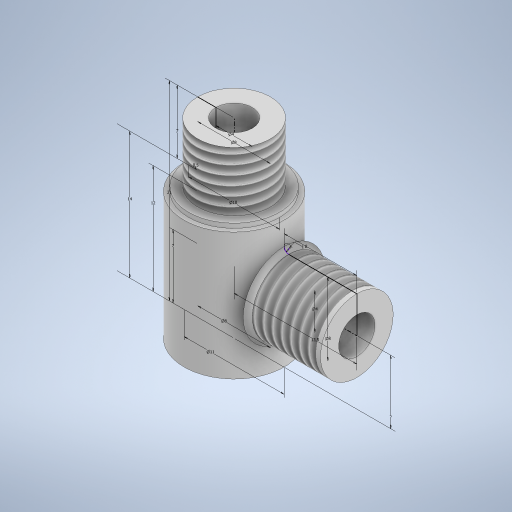
# Autodesk Inventor part: Hudson 1-56
Saved by Autodesk Inventor 2024.2 (Build 282272000, 272)
## iProperties
Created: 2024-10-31
Part Number: Hudson 1-56
Material: Genérico
Document SubType Name: Modeling
Designer: Monica Mora
Density: 1 g/cm^3
Appearance: Valor por defecto
Author: Monica Mora
Autodesk Inventor part; units mm, degrees
ref_plane "YZ Plane" through (0, 0, 0) normal (1, 0, 0) x (0, 1, 0)
ref_plane "XZ Plane" through (0, 0, 0) normal (0, 1, 0) x (-1, 0, 0)
ref_plane "XY Plane" through (0, 0, 0) normal (0, 0, 1) x (1, 0, 0)
sketch "Boceto1" plane through (0, 0, 0) normal (0, 0, 1) x (1, 0, 0)
  line L0 (0, 0) -> (0, 21)
  line L1 (0, 7) -> (13.5, 7)
  line L2 (-2, 21) -> (-4, 21)
  line L3 (-4, 21) -> (-4, 14)
  line L4 (-4, 14) -> (-2, 14)
  line L5 (-2, 21) -> (-2, 14)
  line L6 (-4, 14) -> (-5, 14)
  line L7 (-5, 14) -> (-5, 14.5)
  line L8 (-5, 14.5) -> (-4, 14.5)
  line L9 (-5.5, 0) -> (-5.5, 14)
  line L10 (0, 0) -> (-5.5, 0)
  line L11 (-5, 14) -> (-5.5, 14)
  line L12 (-4, 0) -> (-4, 7)
  line L13 (-4, 7) -> (-4, 12)
  line L14 (-4, 12) -> (-2, 12)
  line L15 (-2, 12) -> (-2, 14)
  line L16 (13.5, 11) -> (6, 11)
  line L17 (13.5, 11) -> (13.5, 9)
  line L18 (13.5, 9) -> (5.5, 9)
  line L19 (5.5, 9) -> (5.5, 11)
  line L20 (13.5, 9) -> (13.5, 7)
  line L21 (5.5, 11) -> (5.5, 11.5)
  arc A0 (5.5, 11.5) -> (6, 11) centre (6, 11.5) ccw
  dimension "d0" = 21
  dimension "d1" = 7
  dimension "d2" = 4
  dimension "d3" = 8
  dimension "d4" = 10
  dimension "d5" = 7
  dimension "d6" = 0.5
  dimension "d7" = 14
  dimension "d8" = 11
  dimension "d9" = 8
  dimension "d10" = 7
  dimension "d11" = 12
  dimension "d12" = 8
  dimension "d13" = 8
  dimension "d14" = 4
  dimension "d17" = 13.5
  dimension "d18" = 1
  constraints: 44 end point, 11 perpendicular, 5 point on line, 5 vertical, 4 horizontal, 2 point on circle, 2 tangent, 1 centre point
  measures "d0" distance of L0.start L0.end
  measures "d1" distance from line of L0.start L1
  measures "d2" diameter of L5 L0
  measures "d3" diameter of L3 L0
  measures "d4" diameter of L7 L0
  measures "d5" distance of L2.end L3.end
  measures "d6" distance between parallel lines of L6 L8
  measures "d7" distance of L9.start L9.end
  measures "d8" diameter of L9 L0
  measures "d9" diameter of L12 L0
  measures "d10" distance of L12.end L12.start
  measures "d11" distance of L13.end L12.start
  measures "d12" diameter of L16 L1
  measures "d13" distance of L16.start L19.end
  measures "d14" diameter of L18 L1
  measures "d17" distance of L1.start L1.end
  measures "d18" diameter of A0
revolve "Revolución1" add sketch "Boceto1" angle 360 about axis through (0, 0, 0) along (0, 1, 0) contours L5 L4 L3 L2 | L15 L14 L13 L12 L10 L9 L11 L6 L4 | L3 L6 L7 L8
revolve "Revolución2" add sketch "Boceto1" angle 360 about axis through (0, 7, 0) along (1, 0, 0) contours L17 L18 L19 L21 A0 L16
thread "Rosca1" size "M8x1" class "6g" standard "ANSI Metric M Profile" length 7
thread "Rosca2" size "M8x1" class "6g" standard "ANSI Metric M Profile" length 7
thread "Rosca3" size "M8x1" class "6H" standard "ANSI Metric M Profile" length 7
